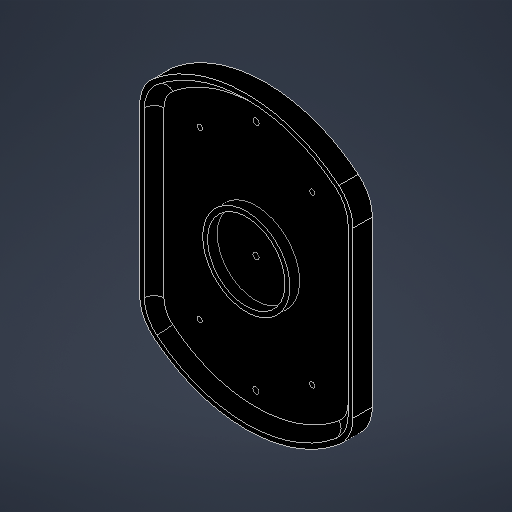
# Autodesk Inventor part: Top Cover
Saved by Autodesk Inventor 2026.1 (Build 301233020, 233B)
## iProperties
Created: 2025-12-02
Part Number: Top Cover
Material: Generic
Document SubType Name: Modeling
Designer: Bahaa
Density: 1 g/cm^3
Appearance: Default(1)
Mass: 80.9788 g
Surface Area: 375.054 cm^2
Volume: 80.9788 cm^3
Mass: 81.1196 g
Surface Area: 374.069 cm^2
Volume: 81.1196 cm^3
Author: Bahaa
Mass: 81.5852 g
Surface Area: 370.413 cm^2
Volume: 81.5852 cm^3
Autodesk Inventor part; units mm, degrees
ref_plane "YZ Plane" through (0, 0, 0) normal (1, 0, 0) x (0, 1, 0)
ref_plane "XZ Plane" through (0, 0, 0) normal (0, 1, 0) x (-1, 0, 0)
ref_plane "XY Plane" through (0, 0, 0) normal (0, 0, 1) x (1, 0, 0)
sketch "Sketch1" plane through (0, 0, 0) normal (0, 1, 0) x (-1, 0, 0)
  circle A0 centre (0, 0) radius 20
  circle A1 centre (0, 0) radius 22.5
  line L0 (-29, -43) -> (29, -43) construction
  line L1 (29, -43) -> (29, 43) construction
  line L2 (29, 43) -> (-29, 43) construction
  line L3 (-29, 43) -> (-29, -43) construction
  line L4 (-29, -43) -> (29, 43) construction
  line L5 (29, -43) -> (-29, 43) construction
  line L6 (0, 0) -> (0, 60) construction
  circle A2 centre (0, 0) radius 75
  line L7 (-75, 0) -> (-55, 0) construction
  line L8 (-55, 0) -> (-55, 50.9902)
  line L9 (-55, 0) -> (-55, -50.9902)
  line L10 (55, 0) -> (55, 50.9902)
  line L11 (55, 0) -> (55, -50.9902)
  circle A3 centre (0, -32.5) radius 15.25
  line L12 (-15.25, -32.5) -> (15.25, -32.5) construction
  line L13 (-5.025, -24.025) -> (5.025, -24.025)
  line L14 (5.025, -24.025) -> (5.025, -20.975)
  line L15 (5.025, -20.975) -> (-5.025, -20.975)
  line L16 (-5.025, -20.975) -> (-5.025, -24.025)
  line L17 (-5.025, -24.025) -> (5.025, -20.975) construction
  line L18 (5.025, -24.025) -> (-5.025, -20.975) construction
  line L19 (-5.025, -40.975) -> (5.025, -40.975)
  line L20 (5.025, -40.975) -> (5.025, -44.025)
  line L21 (5.025, -44.025) -> (-5.025, -44.025)
  line L22 (-5.025, -44.025) -> (-5.025, -40.975)
  line L23 (-5.025, -40.975) -> (5.025, -44.025) construction
  line L24 (5.025, -40.975) -> (-5.025, -44.025) construction
  line L25 (0, -47.75) -> (0, -17.25) construction
  line L26 (0, -75) -> (0, 75) construction
  point P0 (0, -60)
  point P1 (0, -22.5)
  dimension "d0" = 40
  dimension "d1" = 45
  dimension "d2" = 58
  dimension "d3" = 86
  dimension "d4" = 29
  dimension "d5" = 43
  dimension "d26" = 60
  dimension "d35" = 150
  dimension "d36" = 20
  dimension "d37" = 55
  dimension "d67" = 30.5
  dimension "d68" = 32.5
  dimension "d73" = 10.05
  dimension "d74" = 3.05
  dimension "d83" = 20
  constraints: 54 end point, 8 symmetric about line, 6 midpoint, 6 point on circle, 4 centre point, 4 horizontal, 4 parallel, 4 point on line, 3 coincident, 3 perpendicular, 3 vertical
  measures "d0" diameter of A0
  measures "d1" diameter of A1
  measures "d2" distance of L0.start L0.end
  measures "d3" distance of L0.end L1.end
  measures "d4" distance from line of point (0, 0) L1
  measures "d5" distance from line of point (0, 0) L2
  measures "d26" distance of L6.start L6.end
  measures "d35" diameter of A2
  measures "d36" distance of L7.start L7.end
  measures "d37" distance from line of point (0, 0) L8
  measures "d67" diameter of A3
  measures "d68" distance of A0.centre A3.centre
  measures "d73" distance of L15.end L14.end
  measures "d74" distance of L13.end L14.end
  measures "d83" diameter of point (0, -22.5) L12
extrude "Extrusion1" add sketch "Sketch1" along normal blind 5 contours A0 A3 | A0 A3 A1 | A3 A0 | A0 A3 A1 L14 L15 L16 | A1 L16 L13 L14 A3 | L16 L15 L14 A1 | A1 L14 L13 L16 | L10 L11 A2 L9 L8 | L19 L20 L21 L22
hole "Hole1" at (-29, 0, 43) at (29, 0, 43) at (29, 0, -43) at (-29, 0, -43) direction (0, 1, 0) diameter 2.7 end through all
sketch "Sketch2" plane through (0, 5, 0) normal (0, 1, 0) x (1, 0, 0)
  point P0 (0, 0)
hole "Hole2" at (0, 5, 0) direction (0, -1, 0) diameter 3.2 end through all counterbore diameter 5.7 counterbore depth 3
extrude "Extrusion2" add sketch "Sketch1" against normal blind 5 contours A0 A3 A1 | A0 A3 A1 L14 L15 L16 | L16 L15 L14 A1
hole "Hole3" at (0, 0, 60) at (0, 0, -60) direction (0, 1, 0) diameter 3.2 end through all
sketch "Sketch3" plane through (0, 5, 0) normal (0, 1, 0) x (1, 0, 0)
  circle A0 centre (0, -60) radius 1.6 projected
  circle A1 centre (0, 0) radius 2.85 projected
  line L0 (-55, 50.9902) -> (-55, -50.9902) projected
  arc A2 (-55, -50.9902) -> (55, -50.9902) centre (0, 0) ccw projected
  line L1 (55, -50.9902) -> (55, 50.9902) projected
  arc A3 (55, 50.9902) -> (-55, 50.9902) centre (0, 0) ccw projected
  arc A4 (-45, -46.9042) -> (45, -46.9042) centre (0, 0) ccw
  line L2 (-45, -46.9042) -> (-45, 46.9042)
  arc A5 (45, 46.9042) -> (-45, 46.9042) centre (0, 0) ccw
  line L3 (45, 46.9042) -> (45, -46.9042)
  circle A6 centre (0, 0) radius 7.85
  circle A7 centre (29, -43) radius 4.35
  circle A8 centre (-29, -43) radius 4.35
  circle A9 centre (29, 43) radius 4.35
  circle A10 centre (-29, 43) radius 4.35
  line L4 (5, -65) -> (-5, -65)
  line L5 (-5, -65) -> (-5, -55)
  line L6 (-5, -55) -> (5, -55)
  line L7 (5, -55) -> (5, -65)
  line L8 (5, -65) -> (-5, -55) construction
  line L9 (-5, -65) -> (5, -55) construction
  line L10 (5, 65) -> (-5, 65)
  line L11 (-5, 65) -> (-5, 55)
  line L12 (-5, 55) -> (5, 55)
  line L13 (5, 55) -> (5, 65)
  line L14 (5, 65) -> (-5, 55) construction
  line L15 (-5, 65) -> (5, 55) construction
  arc A11 (-42, -45.607) -> (42, -45.607) centre (0, 0) ccw
  line L16 (-42, -45.607) -> (-42, 45.607)
  arc A12 (42, 45.607) -> (-42, 45.607) centre (0, 0) ccw
  line L17 (42, 45.607) -> (42, -45.607)
  arc A13 (-39, -44.2719) -> (39, -44.2719) centre (0, 0) ccw
  line L18 (-39, -44.2719) -> (-39, 44.2719)
  arc A14 (39, 44.2719) -> (-39, 44.2719) centre (0, 0) ccw
  line L19 (39, 44.2719) -> (39, -44.2719)
  arc A15 (-36, -42.8952) -> (36, -42.8952) centre (0, 0) ccw
  line L20 (-36, -42.8952) -> (-36, 42.8952)
  arc A16 (36, 42.8952) -> (-36, 42.8952) centre (0, 0) ccw
  line L21 (36, 42.8952) -> (36, -42.8952)
  line L22 (0, -60) -> (0, 60) construction
  line L23 (25.25, -6.7939) -> (32.483, -4.9011)
  line L24 (32.483, -4.9011) -> (32.483, -5.8267)
  line L25 (32.483, -5.8267) -> (28.0566, -6.9778)
  line L26 (28.0566, -6.9778) -> (32.75, -8.9537)
  line L27 (32.75, -8.9537) -> (28.0328, -10.9415)
  line L28 (28.0328, -10.9415) -> (32.483, -12.1044)
  line L29 (32.483, -12.1044) -> (32.483, -13.0301)
  line L30 (32.483, -13.0301) -> (25.25, -11.1313)
  line L31 (25.25, -11.1313) -> (30.43, -8.9597)
  line L32 (30.43, -8.9597) -> (25.25, -6.7939)
  line L33 (25.2737, -1.335) -> (32.483, 1.9403)
  line L34 (32.483, 1.9403) -> (32.483, 0.9494)
  line L35 (32.483, 0.9494) -> (30.7029, 0.1424)
  line L36 (30.7029, 0.1424) -> (30.7029, -2.8006)
  line L37 (30.7029, -2.8006) -> (32.483, -3.6017)
  line L38 (32.483, -3.6017) -> (32.483, -4.5866)
  line L39 (32.483, -4.5866) -> (25.2737, -1.335)
  line L40 (27.4454, -1.335) -> (29.9138, -2.4446)
  line L41 (29.9138, -2.4446) -> (29.9138, -0.2136)
  line L42 (29.9138, -0.2136) -> (27.4454, -1.335)
  line L43 (25.5407, 2.9608) -> (25.5407, 4.468)
  spline S0 degree 2 poles (25.5407, 4.468) (25.5407, 5.5894) (26.6562, 7.0016) (27.5285, 7.0016) knots 0 0 0 1 2 2 2
  spline S1 degree 2 poles (27.5285, 7.0016) (28.2286, 7.0016) (29.2967, 6.0878) (29.5103, 5.1266) knots 0 0 0 1 2 2 2
  line L44 (29.5103, 5.1266) -> (32.483, 7.1381)
  line L45 (32.483, 7.1381) -> (32.483, 6.0522)
  line L46 (32.483, 6.0522) -> (29.629, 4.1238)
  line L47 (29.629, 4.1238) -> (29.629, 3.9102)
  line L48 (29.629, 3.9102) -> (32.483, 3.9102)
  line L49 (32.483, 3.9102) -> (32.483, 2.9608)
  line L50 (32.483, 2.9608) -> (25.5407, 2.9608)
  line L51 (26.3774, 3.9102) -> (28.7983, 3.9102)
  spline S2 degree 2 poles (28.7983, 3.9102) (28.8398, 6.0107) (27.5819, 6.0107) knots 0 0 0 1 1 1
  spline S3 degree 2 poles (27.5819, 6.0107) (27.1428, 6.0107) (26.5791, 5.5182) (26.3774, 4.6994) (26.3774, 3.9102) knots 0 0 0 1 2 3 3 3
  line L52 (26.3121, 12.6444) -> (26.9292, 11.879)
  spline S4 degree 2 poles (26.9292, 11.879) (26.6147, 11.5704) (26.3002, 11.072) (26.3002, 10.6032) knots 0 0 0 1 2 2 2
  spline S5 degree 2 poles (26.3002, 10.6032) (26.3002, 10.093) (26.7631, 9.4521) (27.125, 9.4521) knots 0 0 0 1 2 2 2
  spline S6 degree 2 poles (27.125, 9.4521) (27.4454, 9.4521) (27.926, 10.0099) (28.5016, 11.3509) (29, 12.0985) (29.5993, 12.5732) (30.2638, 12.8105) (30.6317, 12.8105) knots 0 0 0 1 2 3 4 5 6 6 6
  spline S7 degree 2 poles (30.6317, 12.8105) (31.498, 12.8105) (32.7203, 11.5526) (32.7203, 10.6566) knots 0 0 0 1 2 2 2
  spline S8 degree 2 poles (32.7203, 10.6566) (32.7203, 9.7844) (31.765, 8.4494) (30.8157, 8.0874) knots 0 0 0 1 2 2 2
  line L53 (30.8157, 8.0874) -> (30.5487, 9.0368)
  spline S9 degree 2 poles (30.5487, 9.0368) (31.7176, 9.553) (31.7176, 10.627) knots 0 0 0 1 1 1
  spline S10 degree 2 poles (31.7176, 10.627) (31.7176, 11.1432) (31.1005, 11.8315) (30.6258, 11.8315) knots 0 0 0 1 2 2 2
  spline S11 degree 2 poles (30.6258, 11.8315) (30.341, 11.8315) (29.7714, 11.4695) (29.4035, 10.9296) (28.9229, 9.7607) (28.5253, 9.1317) (27.9735, 8.6748) (27.4276, 8.4612) (27.1191, 8.4612) knots 0 0 0 1 2 3 4 5 6 7 7 7
  spline S12 degree 2 poles (27.1191, 8.4612) (26.3714, 8.4612) (25.3212, 9.6598) (25.3212, 10.5202) knots 0 0 0 1 2 2 2
  spline S13 degree 2 poles (25.3212, 10.5202) (25.3212, 11.0898) (25.8137, 12.2587) (26.3121, 12.6444) knots 0 0 0 1 2 2 2
  point P0 (-5, -64.8074)
  point P1 (-5, -61.7981)
  point P2 (-5, 61.7981)
  point P3 (-5, 64.8074)
  point P4 (5, 64.8074)
  point P5 (5, 61.7981)
  point P6 (5, -61.7981)
  point P7 (5, -64.8074)
  point P8 (5, 58.7878)
  point P9 (5, 55.7763)
  point P10 (5, -55.7763)
  point P11 (5, -58.7878)
  point P12 (-5, -58.7878)
  point P13 (-5, -55.7763)
  point P14 (-5, 55.7763)
  point P15 (-5, 58.7878)
  point P16 (29, 0)
  point P17 (-29, 0)
  point P18 (-30.1381, -47.1985)
  point P19 (-32.4661, -45.6284)
  point P20 (-32.4661, 45.6284)
  point P21 (-30.1381, 47.1985)
  point P22 (30.1381, 47.1985)
  point P23 (32.4661, 45.6284)
  point P24 (32.4661, -45.6284)
  point P25 (30.1381, -47.1985)
  dimension "d0" = 40
  dimension "d1" = 45
  dimension "d2" = 58
  dimension "d3" = 86
  dimension "d4" = 29
  dimension "d5" = 43
  dimension "d26" = 60
  dimension "d35" = 150
  dimension "d36" = 20
  dimension "d37" = 55
  dimension "d67" = 30.5
  dimension "d68" = 32.5
  dimension "d73" = 10.05
  dimension "d74" = 3.05
  dimension "d83" = 20
  dimension "d38" = 10
  dimension "d39" = 5
  dimension "d50" = 10
  dimension "d51" = 10
  dimension "d52" = 10
  dimension "d53" = 10
  dimension "d55" = 3
  dimension "d57" = 3
  dimension "d58" = 3
  dimension "d84" = 29
  dimension "d85" = 29
  constraints: 42 end point, 16 point on circle, 13 centre point, 5 midpoint, 4 parallel, 2 horizontal, 2 horizontal alignment, 2 perpendicular, 1 vertical, 14 other
  measures "d38" radial gap between concentric circles of A2 A4
  measures "d39" radial gap between concentric circles of A1 A6
  measures "d50" distance of L4.end L5.end
  measures "d51" distance of L5.end L6.end
  measures "d52" distance of L11.end L12.end
  measures "d53" distance of L10.end L11.end
  measures "d55" radial gap between concentric circles of A4 A11
  measures "d57" radial gap between concentric circles of A11 A13
  measures "d58" radial gap between concentric circles of A13 A15
  measures "d84" distance of point (29, 0) point (0, 0)
  measures "d85" distance of point (0, 0) point (-29, 0)
extrude "Extrusion3" cut sketch "Sketch3" against normal blind 0.25 contours A11 L17 A12 L13 A5 L3 A4 L7 | L5 A4 L2 A5 L11 A12 L16 A11 | L23 L24 L25 L26 L27 L28 L29 L30 L31 L32 | L33 L34 L35 L36 L37 L38 L39 | L43 S0 S1 L44 L45 L46 L47 L48 L49 L50 | L52 S4 S5 S6 S7 S8 L53 S9 S10 S11 S12 S13
extrude "Extrusion9" cut sketch "Sketch3" against normal blind 0.25 contours A13 L19 A14 L13 A12 L17 A11 L7 | L7 A15 A7 L21 A16 A9 L13 A14 L19 A13 | A13 L18 A14 L11 A16 A10 L20 A15 A8 L5 | L5 A11 L16 A12 L11 A14 L18 A13 | A15 A7 | A8 A15 | A9 A16 | A16 A10 picked at (31.5114, -46.4448) picked at (-31.2527, -46.6193) picked at (31.5114, 46.4448) picked at (-31.5114, 46.4448)
fillet "Fillet1" radius 10 4 edges at (45, 4.875, 46.9042) (-45, 4.875, 46.9042) (45, 4.875, -46.9042) (-45, 4.875, -46.9042)
fillet "Fillet2" radius 20 4 edges at (-55, 2.5, 50.9902) (55, 2.5, 50.9902) (55, 2.5, -50.9902) (-55, 2.5, -50.9902)
fillet "Fillet3" radius 1 4 edges at (5, 4.875, 64.8074) (-5, 4.875, 64.8074) (5, 4.875, -64.8074) (-5, 4.875, -64.8074)
fillet "Fillet4" radius 4 4 edges at (36, 4.875, -42.8952) (-36, 4.875, -42.8952) (-36, 4.875, 42.8952) (36, 4.875, 42.8952)
extrude "Extrusion4" [suppressed]
fillet "Fillet5" [suppressed]
fillet "Fillet6" [suppressed]
sketch "Sketch4" plane through (0, 0, 0) normal (0, -1, 0) x (1, 0, 0)
  circle A0 centre (0, 60) radius 1.6 projected
  arc A1 (-55, -42.4264) -> (-47.7273, -57.8542) centre (-35, -42.4264) ccw projected
  arc A2 (-47.7273, -57.8542) -> (47.7273, -57.8542) centre (0, 0) ccw projected
  arc A3 (47.7273, -57.8542) -> (55, -42.4264) centre (35, -42.4264) ccw projected
  line L0 (55, 42.4264) -> (55, -42.4264) projected
  arc A4 (55, 42.4264) -> (47.7273, 57.8542) centre (35, 42.4264) ccw projected
  arc A5 (47.7273, 57.8542) -> (-47.7273, 57.8542) centre (0, 0) ccw projected
  arc A6 (-47.7273, 57.8542) -> (-55, 42.4264) centre (-35, 42.4264) ccw projected
  line L1 (-55, -42.4264) -> (-55, 42.4264) projected
  circle A7 centre (-29, 43) radius 1.35 projected
  circle A8 centre (29, 43) radius 1.35 projected
  circle A9 centre (29, -43) radius 1.35 projected
  circle A10 centre (-29, -43) radius 1.35 projected
  circle A11 centre (0, 0) radius 22.5 projected
  arc A12 (46.1364, 55.9257) -> (-46.1364, 55.9257) centre (0, 0) ccw
  arc A13 (52.5, 42.4264) -> (46.1364, 55.9257) centre (35, 42.4264) ccw
  line L2 (52.5, 42.4264) -> (52.5, -42.4264)
  arc A14 (46.1364, -55.9257) -> (52.5, -42.4264) centre (35, -42.4264) ccw
  arc A15 (-46.1364, -55.9257) -> (46.1364, -55.9257) centre (0, 0) ccw
  arc A16 (-52.5, -42.4264) -> (-46.1364, -55.9257) centre (-35, -42.4264) ccw
  line L3 (-52.5, -42.4264) -> (-52.5, 42.4264)
  arc A17 (-46.1364, 55.9257) -> (-52.5, 42.4264) centre (-35, 42.4264) ccw
  dimension "d63" = 2.5
  constraints: 12 point on circle, 6 centre point, 4 end point, 7 other
  measures "d63" radial gap between concentric circles of A5 A12
extrude "Extrusion5" add sketch "Sketch4" along normal blind 5 contours L1 A6 A5 A4 L0 A3 A2 A1
fillet "Fillet7" radius 5 8 edges at (-50.8293, 0, 49.8884) (-52.5, 0, 0) (-50.8293, 0, -49.8884) (0, 0, -72.5) (50.8293, 0, -49.8884) (52.5, 0, 0) (50.8293, 0, 49.8884) (0, 0, 72.5)
extrude "Extrusion6" cut sketch "Sketch1" against normal blind 2 from surface at 5 contours A3 A0 | A0 A3 A1 L14 L15 L16 | A1 L16 L13 L14 A3 | L16 L15 L14 A1 | A1 L14 L13 L16 | L19 L20 L21 L22 picked at (0, -18.9956)
extrude "Extrusion7" cut sketch "Sketch1" against normal blind 2 from surface at 3 contours L16 L15 L14 A1 | A1 L14 L13 L16 | L19 L20 L21 L22
extrude "Extrusion8" [suppressed]
chamfer "Chamfer1" distance 2 angle 45 1 edges at (15.25, 5, -32.5)
fillet "Fillet8" [suppressed]
fillet "Fillet9" radius 1 4 edges at (5, 4.875, 55.7763) (-5, 4.875, 55.7763) (5, 4.875, -55.7763) (-5, 4.875, -55.7763)
fillet "Fillet10" [suppressed]
sketch "Sketch5" plane through (0, 5, 0) normal (0, 1, 0) x (1, 0, 0)
  arc A0 (-5, 63.7181) -> (-6.0938, 64.7137) centre (-6, 63.7181) ccw projected
  arc A1 (-6.0938, 64.7137) -> (-41.3636, 50.1403) centre (0, 0) ccw projected
  arc A2 (-41.3636, 50.1403) -> (-45, 42.4264) centre (-35, 42.4264) ccw projected
  line L0 (-45, -42.4264) -> (-45, 42.4264) projected
  arc A3 (-45, -42.4264) -> (-41.3636, -50.1403) centre (-35, -42.4264) ccw projected
  arc A4 (-41.3636, -50.1403) -> (-6.0937, -64.7137) centre (0, 0) ccw projected
  arc A5 (-6.0937, -64.7137) -> (-5, -63.7181) centre (-6, -63.7181) ccw projected
  line L1 (-5, -56.6833) -> (-5, -63.7181) projected
  arc A6 (5, -63.7181) -> (6.0938, -64.7137) centre (6, -63.7181) ccw projected
  arc A7 (6.0938, -64.7137) -> (41.3636, -50.1403) centre (0, 0) ccw projected
  arc A8 (41.3636, -50.1403) -> (45, -42.4264) centre (35, -42.4264) ccw projected
  line L2 (45, 42.4264) -> (45, -42.4264) projected
  arc A9 (45, 42.4264) -> (41.3636, 50.1403) centre (35, 42.4264) ccw projected
  arc A10 (41.3636, 50.1403) -> (6.0937, 64.7137) centre (0, 0) ccw projected
  arc A11 (6.0937, 64.7137) -> (5, 63.7181) centre (6, 63.7181) ccw projected
  line L3 (5, 56.6833) -> (5, 63.7181) projected
  line L4 (26.3121, 12.6444) -> (26.9292, 11.879) projected
  line L5 (30.8157, 8.0874) -> (30.5487, 9.0368) projected
  line L6 (26.3774, 3.9102) -> (28.7983, 3.9102) projected
  line L7 (25.5407, 2.9608) -> (25.5407, 4.468) projected
  line L8 (32.483, 2.9608) -> (25.5407, 2.9608) projected
  line L9 (32.483, 3.9102) -> (32.483, 2.9608) projected
  line L10 (29.629, 3.9102) -> (32.483, 3.9102) projected
  line L11 (29.629, 4.1238) -> (29.629, 3.9102) projected
  line L12 (32.483, 6.0522) -> (29.629, 4.1238) projected
  line L13 (32.483, 7.1381) -> (32.483, 6.0522) projected
  line L14 (29.5103, 5.1266) -> (32.483, 7.1381) projected
  line L15 (29.9138, -2.4446) -> (29.9138, -0.2136) projected
  line L16 (27.4454, -1.335) -> (29.9138, -2.4446) projected
  line L17 (29.9138, -0.2136) -> (27.4454, -1.335) projected
  line L18 (25.2737, -1.335) -> (32.483, 1.9403) projected
  line L19 (32.483, -4.5866) -> (25.2737, -1.335) projected
  line L20 (32.483, -3.6017) -> (32.483, -4.5866) projected
  line L21 (30.7029, -2.8006) -> (32.483, -3.6017) projected
  line L22 (30.7029, 0.1424) -> (30.7029, -2.8006) projected
  line L23 (32.483, 0.9494) -> (30.7029, 0.1424) projected
  line L24 (32.483, 1.9403) -> (32.483, 0.9494) projected
  line L25 (25.25, -6.7939) -> (32.483, -4.9011) projected
  line L26 (30.43, -8.9597) -> (25.25, -6.7939) projected
  line L27 (25.25, -11.1313) -> (30.43, -8.9597) projected
  line L28 (32.483, -13.0301) -> (25.25, -11.1313) projected
  line L29 (32.483, -12.1044) -> (32.483, -13.0301) projected
  line L30 (28.0328, -10.9415) -> (32.483, -12.1044) projected
  line L31 (32.75, -8.9537) -> (28.0328, -10.9415) projected
  line L32 (28.0566, -6.9778) -> (32.75, -8.9537) projected
  line L33 (32.483, -5.8267) -> (28.0566, -6.9778) projected
  line L34 (32.483, -4.9011) -> (32.483, -5.8267) projected
  arc A12 (5, 56.6833) -> (5.8947, 55.6889) centre (6, 56.6833) ccw projected
  arc A13 (34.4615, 44.1407) -> (5.8947, 55.6889) centre (0, 0) ccw projected
  arc A14 (36, 40.9878) -> (34.4615, 44.1407) centre (32, 40.9878) ccw projected
  line L35 (36, -40.9878) -> (36, 40.9878) projected
  arc A15 (34.4615, -44.1407) -> (36, -40.9878) centre (32, -40.9878) ccw projected
  arc A16 (5.8947, -55.6889) -> (34.4615, -44.1407) centre (0, 0) ccw projected
  arc A17 (5.8947, -55.6889) -> (5, -56.6833) centre (6, -56.6833) ccw projected
  line L36 (5, -63.7181) -> (5, -56.6833) projected
  arc A18 (-5.8947, 55.6889) -> (-5, 56.6833) centre (-6, 56.6833) ccw projected
  line L37 (-5, 63.7181) -> (-5, 56.6833) projected
  arc A19 (-5, -56.6833) -> (-5.8947, -55.6889) centre (-6, -56.6833) ccw projected
  arc A20 (-34.4615, -44.1407) -> (-5.8947, -55.6889) centre (0, 0) ccw projected
  arc A21 (-36, -40.9878) -> (-34.4615, -44.1407) centre (-32, -40.9878) ccw projected
  line L38 (-36, 40.9878) -> (-36, -40.9878) projected
  arc A22 (-34.4615, 44.1407) -> (-36, 40.9878) centre (-32, 40.9878) ccw projected
  arc A23 (-5.8947, 55.6889) -> (-34.4615, 44.1407) centre (0, 0) ccw projected
  constraints: 14 other
extrude "Extrusion10" [suppressed]
sketch "Sketch6" plane through (0, 5, 0) normal (0, 1, 0) x (1, 0, 0)
  arc A0 (-5.8947, 55.6889) -> (-5, 56.6833) centre (-6, 56.6833) ccw projected
  line L0 (-5, 57.6888) -> (-5, 56.6833) projected
  arc A1 (-5, 57.6888) -> (-6.1034, 58.6835) centre (-6, 57.6888) ccw projected
  arc A2 (-6.1034, 58.6835) -> (-36.3077, 46.5054) centre (0, 0) ccw projected
  arc A3 (-36.3077, 46.5054) -> (-39, 40.9878) centre (-32, 40.9878) ccw projected
  line L1 (-39, -40.9878) -> (-39, 40.9878) projected
  arc A4 (-39, -40.9878) -> (-36.3077, -46.5054) centre (-32, -40.9878) ccw projected
  arc A5 (-36.3077, -46.5054) -> (-6.1034, -58.6835) centre (0, 0) ccw projected
  arc A6 (-6.1034, -58.6835) -> (-5, -57.6888) centre (-6, -57.6888) ccw projected
  line L2 (-5, -56.6833) -> (-5, -57.6888) projected
  arc A7 (-5, -56.6833) -> (-5.8947, -55.6889) centre (-6, -56.6833) ccw projected
  arc A8 (-34.4615, -44.1407) -> (-5.8947, -55.6889) centre (0, 0) ccw projected
  arc A9 (-36, -40.9878) -> (-34.4615, -44.1407) centre (-32, -40.9878) ccw projected
  line L3 (-36, 40.9878) -> (-36, -40.9878) projected
  arc A10 (-34.4615, 44.1407) -> (-36, 40.9878) centre (-32, 40.9878) ccw projected
  arc A11 (-5.8947, 55.6889) -> (-34.4615, 44.1407) centre (0, 0) ccw projected
  arc A12 (-5, 63.7181) -> (-6.0938, 64.7137) centre (-6, 63.7181) ccw projected
  arc A13 (-6.0938, 64.7137) -> (-41.3636, 50.1403) centre (0, 0) ccw projected
  arc A14 (-41.3636, 50.1403) -> (-45, 42.4264) centre (-35, 42.4264) ccw projected
  line L4 (-45, -42.4264) -> (-45, 42.4264) projected
  arc A15 (-45, -42.4264) -> (-41.3636, -50.1403) centre (-35, -42.4264) ccw projected
  arc A16 (-41.3636, -50.1403) -> (-6.0937, -64.7137) centre (0, 0) ccw projected
  arc A17 (-6.0937, -64.7137) -> (-5, -63.7181) centre (-6, -63.7181) ccw projected
  line L5 (-5, -56.6833) -> (-5, -63.7181) projected
  arc A18 (6.1034, 58.6835) -> (5, 57.6888) centre (6, 57.6888) ccw projected
  line L6 (5, 56.6833) -> (5, 57.6888) projected
  arc A19 (5, 56.6833) -> (5.8947, 55.6889) centre (6, 56.6833) ccw projected
  arc A20 (34.4615, 44.1407) -> (5.8947, 55.6889) centre (0, 0) ccw projected
  arc A21 (36, 40.9878) -> (34.4615, 44.1407) centre (32, 40.9878) ccw projected
  line L7 (36, -40.9878) -> (36, 40.9878) projected
  arc A22 (34.4615, -44.1407) -> (36, -40.9878) centre (32, -40.9878) ccw projected
  arc A23 (5.8947, -55.6889) -> (34.4615, -44.1407) centre (0, 0) ccw projected
  arc A24 (5.8947, -55.6889) -> (5, -56.6833) centre (6, -56.6833) ccw projected
  line L8 (5, -57.6888) -> (5, -56.6833) projected
  arc A25 (5, -57.6888) -> (6.1034, -58.6835) centre (6, -57.6888) ccw projected
  arc A26 (6.1034, -58.6835) -> (36.3077, -46.5054) centre (0, 0) ccw projected
  arc A27 (36.3077, -46.5054) -> (39, -40.9878) centre (32, -40.9878) ccw projected
  line L9 (39, 40.9878) -> (39, -40.9878) projected
  arc A28 (39, 40.9878) -> (36.3077, 46.5054) centre (32, 40.9878) ccw projected
  arc A29 (36.3077, 46.5054) -> (6.1034, 58.6835) centre (0, 0) ccw projected
  line L10 (-26.2913, 9.2178) -> (-26.9084, 9.9832) projected
  line L11 (-30.7949, 13.7747) -> (-30.5279, 12.8254) projected
  line L12 (-25.52, 7.9005) -> (-25.52, 6.963) projected
  line L13 (-32.4622, 7.9005) -> (-25.52, 7.9005) projected
  line L14 (-32.4622, 6.963) -> (-32.4622, 7.9005) projected
  line L15 (-25.52, 6.963) -> (-32.4622, 6.963) projected
  line L16 (-26.3566, 4.3404) -> (-28.7775, 4.3404) projected
  line L17 (-25.52, 5.2898) -> (-25.52, 3.7826) projected
  line L18 (-32.4622, 5.2898) -> (-25.52, 5.2898) projected
  line L19 (-32.4622, 4.3404) -> (-32.4622, 5.2898) projected
  line L20 (-29.6082, 4.3404) -> (-32.4622, 4.3404) projected
  line L21 (-29.6082, 4.1268) -> (-29.6082, 4.3404) projected
  line L22 (-32.4622, 2.1984) -> (-29.6082, 4.1268) projected
  line L23 (-32.4622, 1.1125) -> (-32.4622, 2.1984) projected
  line L24 (-29.4895, 3.124) -> (-32.4622, 1.1125) projected
  line L25 (-25.52, -0.1276) -> (-25.52, -1.0651) projected
  line L26 (-32.4622, -0.1276) -> (-25.52, -0.1276) projected
  line L27 (-32.4622, -1.0651) -> (-32.4622, -0.1276) projected
  line L28 (-25.52, -1.0651) -> (-32.4622, -1.0651) projected
  line L29 (-29.6438, -2.5603) -> (-25.5318, -2.5603) projected
  line L30 (-25.5318, -2.5603) -> (-25.5318, -3.5097) projected
  line L31 (-29.6438, -2.5603) -> (-25.5318, -2.5603) projected
  line L32 (-25.5318, -7.948) -> (-29.8989, -7.948) projected
  line L33 (-25.5318, -6.9986) -> (-25.5318, -7.948) projected
  line L34 (-29.9642, -6.9986) -> (-25.5318, -6.9986) projected
  line L35 (-25.5318, -3.5097) -> (-29.804, -3.5097) projected
  line L36 (-26.2913, -13.5789) -> (-26.9084, -12.8135) projected
  line L37 (-30.7949, -9.022) -> (-30.5279, -9.9713) projected
  arc A30 (-5, 63.7181) -> (-6.0938, 64.7137) centre (-6, 63.7181) ccw projected
  arc A31 (-6.0938, 64.7137) -> (-41.3636, 50.1403) centre (0, 0) ccw projected
  arc A32 (-41.3636, 50.1403) -> (-45, 42.4264) centre (-35, 42.4264) ccw projected
  line L38 (-45, -42.4264) -> (-45, 42.4264) projected
  arc A33 (-45, -42.4264) -> (-41.3636, -50.1403) centre (-35, -42.4264) ccw projected
  arc A34 (-41.3636, -50.1403) -> (-6.0937, -64.7137) centre (0, 0) ccw projected
  arc A35 (-6.0937, -64.7137) -> (-5, -63.7181) centre (-6, -63.7181) ccw projected
  line L39 (-5, -56.6833) -> (-5, -63.7181) projected
  arc A36 (-5.8947, 55.6889) -> (-5, 56.6833) centre (-6, 56.6833) ccw projected
  line L40 (-5, 63.7181) -> (-5, 56.6833) projected
  arc A37 (-5, -56.6833) -> (-5.8947, -55.6889) centre (-6, -56.6833) ccw projected
  arc A38 (-34.4615, -44.1407) -> (-5.8947, -55.6889) centre (0, 0) ccw projected
  arc A39 (-36, -40.9878) -> (-34.4615, -44.1407) centre (-32, -40.9878) ccw projected
  line L41 (-36, 40.9878) -> (-36, -40.9878) projected
  arc A40 (-34.4615, 44.1407) -> (-36, 40.9878) centre (-32, 40.9878) ccw projected
  arc A41 (-5.8947, 55.6889) -> (-34.4615, 44.1407) centre (0, 0) ccw projected
  arc A42 (-5.8947, 55.6889) -> (-5, 56.6833) centre (-6, 56.6833) ccw projected
  line L42 (-5, 63.7181) -> (-5, 56.6833) projected
  arc A43 (-5, -56.6833) -> (-5.8947, -55.6889) centre (-6, -56.6833) ccw projected
  arc A44 (-34.4615, -44.1407) -> (-5.8947, -55.6889) centre (0, 0) ccw projected
  arc A45 (-36, -40.9878) -> (-34.4615, -44.1407) centre (-32, -40.9878) ccw projected
  line L43 (-36, 40.9878) -> (-36, -40.9878) projected
  arc A46 (-34.4615, 44.1407) -> (-36, 40.9878) centre (-32, 40.9878) ccw projected
  arc A47 (-5.8947, 55.6889) -> (-34.4615, 44.1407) centre (0, 0) ccw projected
  constraints: 28 other
extrude "Extrusion11" [suppressed]
equation "\"d37\" = 0.5 * d35 - d36"
equation "\"d51\" = d50"
equation "\"d52\" = d50"
equation "\"d53\" = d50"
body "Solid1"
